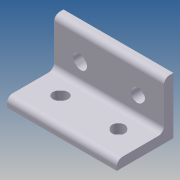
# Autodesk Inventor part: 28-604
Saved by Autodesk Inventor 2011 SP1 (Build 150282100, 282)
## iProperties
Created: 2010-12-09
Part Number: 28-604
Material: Aluminum-6061
Document SubType Name: Modeling
Designer: dc85560
Stock Number: 28-604
Mass: 83.7328 g
Surface Area: 120.004 cm^2
Volume: 30.8977 cm^3
Density: 2.71 g/cm^3
Title: SMART Economy Gusset 80/3"
Author: dc85560
Autodesk Inventor part; units mm, degrees
ref_plane "YZ Plane" through (0, 0, 0) normal (1, 0, 0) x (0, 1, 0)
sketch "Sketch1" plane through (0, 0, 0) normal (0, 0, 1) x (1, 0, 0)
  line L0 (-19.05, 19.05) -> (19.05, 19.05)
  line L1 (19.05, 19.05) -> (19.05, -19.05)
  line L2 (19.05, -19.05) -> (-19.05, -19.05)
  line L3 (-19.05, -19.05) -> (-19.05, 19.05)
  point P0 (0, 0)
  dimension "d0" = 38.1
  dimension "d1" = 38.1
  dimension "d2" = 19.05
  dimension "d3" = 19.05
  constraints: 8 end point, 2 parallel, 1 horizontal, 1 perpendicular
  measures "d0" distance of L0.start L0.end
  measures "d1" distance of L0.end L1.end
  measures "d2" distance from line of point (0, 0) L0
  measures "d3" distance from line of point (0, 0) L3
extrude "Extrusion1" add sketch "Sketch1" against normal blind 74
sketch "Sketch2" plane through (0, 0, 0) normal (0, 0, 1) x (1, 0, 0)
  line L0 (19.05, -19.05) -> (-19.05, -19.05) projected
  line L1 (19.05, 19.05) -> (19.05, -19.05) projected
  line L2 (-19.05, 19.05) -> (12.7, 19.05)
  line L3 (12.7, 19.05) -> (12.7, -12.7)
  line L4 (12.7, -12.7) -> (-19.05, -12.7)
  line L5 (-19.05, -12.7) -> (-19.05, 19.05)
  dimension "d6" = 6.35
  dimension "d7" = 6.35
  constraints: 8 end point, 2 parallel, 1 horizontal, 1 perpendicular
  measures "d6" distance between parallel lines of L3 L1
  measures "d7" distance between parallel lines of L4 L0
extrude "Extrusion2" cut sketch "Sketch2" against normal through all
ref_plane "Work Plane1" through (0, 0, -37) normal (0, 0, 1) x (1, 0, 0)
fillet "Fillet1" radius 3.81 3 edges at (12.7, 19.05, -37) (-19.05, -12.7, -37) (12.7, -12.7, -37)
ref_plane "Work Plane2" through (19.05, -19.05, 0) normal (-0.7071, -0.7071, 0) x (0, 0, -1)
sketch "Sketch7" plane through (12.7, -8.89, 0) normal (-1, 0, 0) x (0, 0, 1)
  line L0 (0, -10.16) -> (-74, -10.16) projected
  line L1 (0, -10.16) -> (-74, -10.16) projected
  line L2 (-37, 35.56) -> (-37, -17.78) projected
  point P0 (-17, 9.84)
  point P1 (-17.95, 8.89)
  dimension "d29" = 20
  dimension "d30" = 19.05
  dimension "d31" = 20
  dimension "d32" = 19.05
  measures "d29" distance from line of point (-17, 9.84) L2
  measures "d30" distance from line of point (-17.95, 8.89) L2
  measures "d31" distance from line of point (-17, 9.84) L0
  measures "d32" distance from line of point (-17.95, 8.89) L0
hole "Hole2" at (12.7, 0.95, -17) at (12.7, 0, -17.95) direction (1, 0, 0) diameter 8.4 end through all clearance for "Socket Head Cap Screw" size "M8" standard "Ansi Metric M Profile"
mirror "Mirror4" about plane through (0, 0, -37) normal (0, 0, 1) of "Hole2"
mirror "Mirror5" about plane through (19.05, -19.05, 0) normal (-0.7071, -0.7071, 0) of "Hole2", "Mirror4"
sketch "Sketch9" plane through (12.7, -8.89, 0) normal (-1, 0, 0) x (0, 0, 1)
  arc A0 (-20.4066, 12.2966) -> (-14.5434, 6.4334) centre (-17.95, 8.89) ccw projected
  arc A1 (-14.5434, 6.4334) -> (-20.4066, 12.2966) centre (-17, 9.84) ccw projected
  line L0 (-19.9698, 12.8098) -> (-20.9198, 11.8598)
  line L1 (-14.9802, 5.9202) -> (-14.0302, 6.8702)
  constraints: 4 end point, 4 point on circle, 4 tangent
extrude "Extrusion7" cut sketch "Sketch9" against normal through all contours A0 L0 A1 | A0 A1 L1
mirror "Mirror6" about plane through (0, 0, -37) normal (0, 0, 1) of "Extrusion7"
mirror "Mirror7" about plane through (19.05, -19.05, 0) normal (-0.7071, -0.7071, 0) of "Extrusion7", "Mirror6"
equation "\"d1\" = d0"
equation "\"d2\" = 0.5 * d1"
equation "\"d3\" = d2"
equation "\"d7\" = d6"
equation "\"d31\" = d29"
equation "\"d32\" = d30"
body "Solid1"
